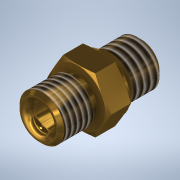
# Autodesk Inventor part: MINI-male-threaded-fitting
Saved by Autodesk Inventor 2021 (Build 250183000, 183)
## iProperties
Company: Prusa Development a.s.
Created: 2019-10-03
Material: Všeobecné
Document SubType Name: Modeling
Density: 1 g/cm^3
Appearance: Mosaz – leštěná
Project: ORIGINAL PRUSA MINI
Authority: Ing. Robert Turinský
Author: ing. Robert Turinský
Revision Number: R4
Autodesk Inventor part; units mm, degrees
ref_plane "YZ Plane" through (0, 0, 0) normal (1, 0, 0) x (0, 1, 0)
ref_plane "XZ Plane" through (0, 0, 0) normal (0, 1, 0) x (-1, 0, 0)
sketch "Náčrt1" plane through (0, 0, 0) normal (0, 1, 0) x (-1, 0, 0)
  line L0 (0, -3.7408) -> (0, 22.4445) projected
  line L1 (9, 0) -> (-1.5, 0) projected
  line L2 (2.05, 0.3) -> (2.05, 7)
  line L3 (2.05, 7) -> (1.1, 7.5485)
  line L4 (1.1, 7.5485) -> (1.1, 11.6515)
  line L5 (1.1, 11.6515) -> (2.05, 12.2)
  line L6 (2.05, 12.2) -> (2.05, 17.0814)
  arc A0 (3.2, 18.5) -> (2.05, 17.0814) centre (3.5, 17.0814) ccw
  line L7 (3.2, 18.5) -> (3.4, 18.5)
  line L8 (3.4, 18.5) -> (4, 17.9)
  line L9 (4, 17.9) -> (4, 12.65)
  line L10 (4, 12.65) -> (3.375, 12.65)
  line L11 (3.375, 12.65) -> (3.375, 11.4)
  line L12 (3.375, 11.4) -> (5, 11.4)
  line L13 (5, 11.4) -> (5, 6.9)
  line L14 (5, 6.9) -> (3.2, 6.9)
  line L15 (3.2, 6.9) -> (3.2, 5.65)
  line L16 (3.2, 5.65) -> (4, 5.65)
  line L17 (4, 5.65) -> (4, 0.75)
  line L18 (4, 0.75) -> (3.25, 0)
  line L19 (3.25, 0) -> (2.35, 0)
  line L20 (2.05, 0.3) -> (2.35, 0)
  line L21 (5, 11.4) -> (7.5, 10.7301)
  line L22 (7.5, 10.7301) -> (7.5, 11.4)
  line L23 (7.5, 11.4) -> (5, 11.4)
  line L24 (7.5, 6.9) -> (5, 6.9)
  line L25 (7.5, 6.9) -> (5, 6.9)
  line L26 (5, 6.9) -> (5, 7.4)
  line L27 (7.5, 6.9) -> (7.5, 8.1034)
  line L28 (7.5, 8.1034) -> (4.875, 7.4)
  line L29 (4.875, 7.4) -> (4.875, 6.9)
  line L30 (4.875, 6.9) -> (7.5, 6.9)
  line L31 (7.5, 10.7301) -> (7.5, 10.6966)
  line L32 (7.5, 10.6966) -> (4.875, 11.4)
  point P0 (0, 0)
  point P1 (5, 7.4335)
  dimension "d0" = 4.1
  dimension "d1" = 2.2
  dimension "d3" = 60
  dimension "d4" = 60
  dimension "d5" = 0.3
  dimension "d6" = 45
  dimension "d7" = 8
  dimension "d8" = 0.75
  dimension "d9" = 1.45
  dimension "d11" = 1.25
  dimension "d12" = 6.4
  dimension "d13" = 18.5
  dimension "d14" = 6.3
  dimension "d15" = 6.75
  dimension "d16" = 10
  dimension "d17" = 7
  dimension "d18" = 1.25
  dimension "d19" = 7.1
  dimension "d20" = 0.6
  dimension "d21" = 6.4
  dimension "d22" = 4.5
  dimension "d32" = 15
  dimension "d33" = 15
  dimension "d35" = 10
  dimension "d38" = 15
  dimension "d39" = 9.75
  dimension "d40" = 0.5
  constraints: 62 end point, 13 perpendicular, 6 point on line, 5 collinear, 4 vertical, 3 parallel, 2 horizontal, 2 point on circle, 1 centre point, 1 tangent, 1 vertical alignment
  measures "d0" diameter of L6 L0
  measures "d1" diameter of L4 L0
  measures "d3" angle of L0 L5
  measures "d4" angle of L0 L3
  measures "d5" horizontal distance of L2.start L19.end
  measures "d6" angle of L1 L20
  measures "d7" diameter of L17 L0
  measures "d8" horizontal distance of L17.end L18.end
  measures "d9" radius of A0
  measures "d11" distance of L14.end L15.end
  measures "d12" diameter of L15 L0
  measures "d13" distance between parallel lines of L1 L7
  measures "d14" distance from line of L5.end L7
  measures "d15" diameter of L11 L0
  measures "d16" diameter of L13 L0
  measures "d17" distance from line of L19 L2.end
  measures "d18" distance of L10.end L11.end
  measures "d19" distance between parallel lines of L12 L7
  measures "d20" horizontal distance of L7.end L8.end
  measures "d21" diameter of L7.start L0
  measures "d22" distance of L12.end L13.end
  measures "d32" diameter of L22 L0
  measures "d33" angle of L23 L21
  measures "d35" diameter of L26 L0
  measures "d38" angle of L30 L28
  measures "d39" diameter of L29 L0
  measures "d40" distance of L28.end L29.end
revolve "Rotace1" add sketch "Náčrt1" angle 360 about axis through (0, 0, -10) along (0, 0, 1) contours L1 L20 L2 L3 L4 L5 L6 A0 L7 L8 L9 L10 L11 L12 L32 L13 L28 L29 L14 L15 L16 L17 L18 | L29 L28 L13 L14 | L32 L12 L13
thread "Závit1" size "M8x1.25" class "6g" standard "ANSI Metric M Profile" full length
thread "Závit2" size "M8x1" class "6g" standard "ANSI Metric M Profile" full length
ref_plane "Pracovní rovina1" through (0, 0, 6.9) normal (0, 0, 1) x (1, 0, 0)
sketch "Náčrt2" plane through (0, 0, 6.9) normal (0, 0, 1) x (1, 0, 0)
  circle A0 centre (0, 0) radius 3.2 projected
  circle A1 centre (0, 0) radius 5 projected
  line L0 (-5.7735, 0) -> (-2.8868, 5)
  line L1 (-2.8868, 5) -> (2.8868, 5)
  line L2 (2.8868, 5) -> (5.7735, 0)
  line L3 (5.7735, 0) -> (2.8868, -5)
  line L4 (2.8868, -5) -> (-2.8868, -5)
  line L5 (-2.8868, -5) -> (-5.7735, 0)
  dimension "d29" = 10
  constraints: 12 end point, 1 coincident, 1 horizontal, 13 other
  measures "d29" distance between parallel lines of L4 L1
extrude "Vysunutí1" add sketch "Náčrt2" along normal blind 4.5
revolve "Rotace2" cut sketch "Náčrt1" angle 360 about axis through (0, 0, -10) along (0, 0, 1) contours L32 L12 L13 | L13 L21 L31 L32 | L23 L22 L21
revolve "Rotace3" cut sketch "Náčrt1" angle 360 about axis through (0, 0, -10) along (0, 0, 1) contours L29 L28 L13 L14 | L13 L28 L27 L24
equation "\"d30\" = d22"
equation "\"d4\" = d3"
equation "\"d38\" = d33"
equation "\"d28\" = -d19 + d13 - d22"
